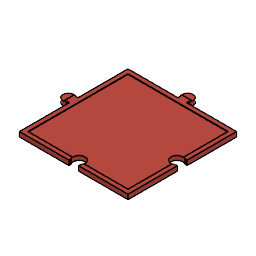
Kidslab Platte - Outside Marker v2 (Autodesk Fusion 360 design; units mm, degrees)
Autodesk Fusion 360 part; units mm, degrees
note: some values were not read from the file. Set by a fixed rule: which face or edge a step refers to.
box "Grundkörper Quader1" add length 50 width 50 height 2 placed x (0, 0, 1) y (1, 0, 0) z (0, 1, 0) at (0, 0, 0) makes body 1
sketch "Skizze5" plane through (0, 2, 0) normal (0, 1, 0) x (-1, 0, 0)
  line L0 (0, 50) -> (-50, 50)
  line L1 (-50, 50) -> (-50, 0)
  line L2 (-50, 0) -> (0, 0)
  line L3 (0, 0) -> (0, 50)
  line L4 (-25, 0) -> (-25, 50) construction
  line L5 (-23, 0) -> (-23, -0.6972)
  line L6 (-27, 0) -> (-27, -0.6972)
  arc A0 (-27.1429, -1.2123) -> (-22.8571, -1.2123) centre (-25, -2.5) ccw
  arc A1 (-27.1429, -1.2123) -> (-27, -0.6972) centre (-28, -0.6972) ccw
  arc A2 (-23, -0.6972) -> (-22.8571, -1.2123) centre (-22, -0.6972) ccw
  point P0 (-23, 3)
  dimension "d27" = 5
  dimension "d28" = 2
  dimension "d30" = 3
  constraint midpoint L2 L4.start
  constraint midpoint L0 L4.end
  constraint coincident L2 L5.start
  constraint perpendicular L2 L5
  constraint vertical L4.start A0.centre
  constraint symmetric L4 L5.start L6.start
  constraint tangent L6 A1
  constraint tangent A0 A1
  constraint tangent L5 A2
  constraint tangent A0 A2
  measures "d27" diameter of A0
  measures "d28" distance of L4 L5
  measures "d30" distance of L5.start P0
extrude "Extrusion4" add sketch "Skizze5" against normal blind 2 separate body contours L2 L5 L6 A0 A1 A2 makes body 2
sketch "Skizze7" plane through (0, 2, 0) normal (0, 1, 0) x (-1, 0, 0)
  line L0 (0, 50) -> (-50, 50)
  line L1 (-50, 50) -> (-50, 0)
  line L2 (-50, 0) -> (0, 0)
  line L3 (0, 0) -> (0, 50)
  line L4 (-25, 0) -> (-25, 50) construction
  line L5 (-50, 25) -> (0, 25) construction
  point P0 (-25, 25)
  constraint midpoint L2 L4.start
  constraint midpoint L0 L4.end
  constraint midpoint L1 L5.start
  constraint midpoint L3 L5.end
  constraint midpoint L4 P0
pattern_circular "C-Anordnung1" count 4 over 360 about axis through (25, -48, 25) along (0, 1, 0) of bodies 2 makes body 3 at (-1.4261, 0.6667, 27.2576) makes body 4 at (22.6104, 0.6667, 51.7651) makes body 5 at (51.7651, 0.6667, 27.3896)
mirror "Spiegeln3" about plane through (0, 0, 50) normal (0, 0, 1) of bodies 4 makes body 6
mirror "Spiegeln4" about plane through (50, 0, 0) normal (1, 0, 0) of bodies 5 makes body 7
combine "Kombinieren2" operation add target body 1 tool bodies 3 2
combine "Kombinieren3" operation cut target body 1 tool bodies 6 7
move_face "Flächen versetzen1" offset -0.2 10 faces at (48.2349, 0.6667, 27.3896) (22.6104, 0.6667, 48.2349) (23, 1.3333, 49.7676) (22.8795, 1.3333, 48.8269) (27.001, 1.3333, 49.2577) (27, 1.3333, 49.7676) (49.7676, 1.3333, 23) (48.8269, 0.6667, 22.8795) (49.7676, 1.3333, 27) (49.2577, 0.6667, 27.001) on bodies 1
delete_body "Körper entfernen1" bodies 4
delete_body "Körper entfernen2" bodies 5
sketch "Skizze8" plane through (0, 2, 0) normal (0, 1, 0) x (-1, 0, 0)
  line L0 (-49.3028, 22.8) -> (-50, 22.8)
  line L1 (-50, 22.8) -> (-50, 0)
  line L2 (-50, 0) -> (-27, 0)
  line L3 (-27, 0) -> (-27, -0.6972)
  arc A0 (-27.1429, -1.2123) -> (-27, -0.6972) centre (-28, -0.6972) ccw
  arc A1 (-27.1429, -1.2123) -> (-22.8571, -1.2123) centre (-25, -2.5) ccw
  arc A2 (-23, -0.6972) -> (-22.8571, -1.2123) centre (-22, -0.6972) ccw
  line L4 (-23, -0.6972) -> (-23, 0)
  line L5 (-23, 0) -> (0, 0)
  line L6 (0, 0) -> (0, 23)
  line L7 (0, 23) -> (0.6972, 23)
  arc A3 (1.2123, 22.8571) -> (0.6972, 23) centre (0.6972, 22) ccw
  arc A4 (1.2123, 22.8571) -> (1.2123, 27.1429) centre (2.5, 25) ccw
  arc A5 (0.6972, 27) -> (1.2123, 27.1429) centre (0.6972, 28) ccw
  line L8 (0.6972, 27) -> (0, 27)
  line L9 (0, 27) -> (0, 50)
  line L10 (0, 50) -> (-22.8, 50)
  line L11 (-22.8, 50) -> (-22.8, 49.3028)
  arc A6 (-22.8, 49.3028) -> (-22.6857, 48.8907) centre (-22, 49.3028) ccw
  arc A7 (-27.3143, 48.8907) -> (-22.6857, 48.8907) centre (-25, 47.5) ccw
  arc A8 (-27.3143, 48.8907) -> (-27.2, 49.3028) centre (-28, 49.3028) ccw
  line L12 (-27.2, 49.3028) -> (-27.2, 50)
  line L13 (-27.2, 50) -> (-50, 50)
  line L14 (-50, 50) -> (-50, 27.2)
  line L15 (-50, 27.2) -> (-49.3028, 27.2)
  arc A9 (-49.3028, 27.2) -> (-48.8907, 27.3143) centre (-49.3028, 28) ccw
  arc A10 (-48.8907, 22.6857) -> (-48.8907, 27.3143) centre (-47.5, 25) ccw
  arc A11 (-48.8907, 22.6857) -> (-49.3028, 22.8) centre (-49.3028, 22) ccw
  line L16 (-2, 2) -> (-48, 2)
  line L17 (-48, 2) -> (-48, 48)
  line L18 (-48, 48) -> (-2, 48)
  line L19 (-2, 48) -> (-2, 2)
  line L20 (2, -2) -> (-52, -2)
  line L21 (-52, -2) -> (-52, 52)
  line L22 (-52, 52) -> (2, 52)
  line L23 (2, 52) -> (2, -2)
  line L24 (0, 0) -> (0, 50)
  line L25 (0, 50) -> (-50, 50)
  line L26 (-50, 50) -> (-50, 0)
  line L27 (-50, 0) -> (0, 0)
  dimension "d42" = 2
  dimension "d43" = 2
  dimension "d45" = 2
  dimension "d46" = 2
  dimension "d47" = 2
  dimension "d48" = 2
  dimension "d49" = 2
  dimension "d50" = 2
  constraint horizontal L16
  constraint vertical L17
  constraint horizontal L18
  constraint vertical L19
  constraint horizontal L20
  constraint vertical L21
  constraint horizontal L22
  constraint vertical L23
  measures "d42" distance of L5 L16
  measures "d43" distance of L1 L17
  measures "d45" distance of L19 L24
  measures "d46" distance of L18 L25
  measures "d47" distance of L23 L24
  measures "d48" distance of L21 L26
  measures "d49" distance of L20 L27
  measures "d50" distance of L10 L22
extrude "Extrusion5" add sketch "Skizze8" along normal blind 0.2 contours L0 L1 L2 L5 L6 L9 L10 L11 A6 A7 A10 A11 L16 L17 L18 L19 L24 L25 L26 L27 | A7 A8 L12 L13 L14 L15 A9 A10 L17 L18 L25 L26 | L3 A0 A1 A2 L4 L20 L27 | L7 A3 A4 A5 L8 L23 L24 bodies 1
equation "d5 = StärkeFläche"
equation "Magnet_Durchmesser = 5 mm"
equation "Magnet_Stärke = 1.5 mm"
equation "Halterung_Breite = 5.5 mm"
equation "StärkeFläche = 2 mm"
equation "d32 = -StärkeFläche"
equation "d40 = Threshold"
equation "Threshold = -0.2 mm"
equation "d42 = MarkerAbstand"
equation "d43 = MarkerAbstand"
equation "MarkerAbstand = 2 mm"
equation "d45 = MarkerAbstand"
equation "d46 = MarkerAbstand"
equation "d47 = MarkerAbstand"
equation "d48 = MarkerAbstand"
equation "d49 = MarkerAbstand"
equation "d50 = MarkerAbstand"
equation "MarkerHöhe = 0.2 mm"
equation "d52 = MarkerHöhe"
named bodies: "Platte", "Puzzleteil", "Puzzleteil (1)", "Puzzleteil (2)", "Puzzleteil (3)", "Puzzleteil (2) (1)", "Puzzleteil (3) (1)"
